Autodesk Fusion 360 part; units mm, degrees
(part 3 of 6)
  spline S86 degree 5 poles (-25.5634, -29.6746) (-25.5637, -29.6656) (-25.5642, -29.6475) (-25.565, -29.6203) (-25.5662, -29.5841) (-25.5679, -29.5389) (-25.5697, -29.4938) (-25.5716, -29.4487) (-25.5738, -29.4036) (-25.576, -29.3586) (-25.5785, -29.3137) (-25.581, -29.2688) (-25.5838, -29.2239) (-25.5867, -29.1791) (-25.5897, -29.1343) (-25.5929, -29.0896) (-25.5963, -29.045) (-25.5998, -29.0004) (-25.6035, -28.9558) (-25.6074, -28.9113) (-25.6114, -28.8669) (-25.6156, -28.8225) (-25.62, -28.7782) (-25.6245, -28.7339) (-25.6292, -28.6897) (-25.6341, -28.6456) (-25.6391, -28.6015) (-25.6443, -28.5575) (-25.6497, -28.5135) (-25.6553, -28.4696) (-25.661, -28.4258) (-25.667, -28.382) (-25.6731, -28.3383) (-25.6794, -28.2947) (-25.6858, -28.2511) (-25.6925, -28.2076) (-25.6993, -28.1642) (-25.7064, -28.1208) (-25.7136, -28.0775) (-25.721, -28.0343) (-25.7287, -27.9912) (-25.7365, -27.9482) (-25.7445, -27.9052) (-25.7527, -27.8623) (-25.7612, -27.8195) (-25.7698, -27.7767) (-25.7773, -27.7409) (-25.7831, -27.7135) (-25.7871, -27.6947) (-25.7894, -27.6845) (-25.7898, -27.6827) knots -1 -1 -1 -1 -1 -1 -0.985714 -0.971429 -0.957143 -0.942857 -0.928571 -0.914286 -0.9 -0.885714 -0.871429 -0.857143 -0.842857 -0.828571 -0.814286 -0.8 -0.785714 -0.771429 -0.757143 -0.742857 -0.728571 -0.714286 -0.7 -0.685714 -0.671429 -0.657143 -0.642857 -0.628571 -0.614286 -0.6 -0.585714 -0.571429 -0.557143 -0.542857 -0.528571 -0.514286 -0.5 -0.485714 -0.471429 -0.457143 -0.442857 -0.428571 -0.414286 -0.4 -0.385714 -0.371429 -0.357143 -0.354152 -0.354152 -0.354152 -0.354152 -0.354152 -0.354152
  spline S87 degree 3 poles (-25.5364, -27.1352) (-25.5938, -27.1658) (-25.6448, -27.2073) (-25.7278, -27.3076) (-25.7591, -27.3654) (-25.7914, -27.4687) (-25.7988, -27.5113) (-25.8026, -27.5975) (-25.7989, -27.6406) (-25.7898, -27.6827) knots 0 0 0 0 0.019532 0.019532 0.039064 0.039064 0.051994 0.051994 0.064924 0.064924 0.064924 0.064924
  arc A44 (-25.5364, -27.1352) -> (-25.4617, -27.0952) centre (-40, 0) ccw
  spline S88 degree 3 poles (-24.8656, -27.1885) (-24.9108, -27.1416) (-24.9648, -27.1041) (-25.084, -27.0518) (-25.1482, -27.0375) (-25.2564, -27.0349) (-25.2994, -27.0394) (-25.3832, -27.0594) (-25.4237, -27.0748) (-25.4617, -27.0952) knots 0 0 0 0 0.019532 0.019532 0.039064 0.039064 0.051994 0.051994 0.064924 0.064924 0.064924 0.064924
  spline S89 degree 5 poles (-24.8656, -27.1885) (-24.8643, -27.1898) (-24.857, -27.1973) (-24.8437, -27.2111) (-24.8242, -27.2311) (-24.7984, -27.2573) (-24.7677, -27.2882) (-24.7368, -27.319) (-24.7057, -27.3496) (-24.6744, -27.3802) (-24.6429, -27.4106) (-24.6113, -27.4409) (-24.5795, -27.471) (-24.5475, -27.5011) (-24.5154, -27.531) (-24.483, -27.5608) (-24.4506, -27.5905) (-24.4179, -27.6201) (-24.3851, -27.6495) (-24.3522, -27.6789) (-24.319, -27.7081) (-24.2858, -27.7372) (-24.2523, -27.7662) (-24.2188, -27.7951) (-24.1851, -27.8239) (-24.1512, -27.8526) (-24.1172, -27.8811) (-24.083, -27.9096) (-24.0487, -27.9379) (-24.0143, -27.9661) (-23.9797, -27.9943) (-23.945, -28.0223) (-23.9101, -28.0502) (-23.8751, -28.078) (-23.84, -28.1057) (-23.8047, -28.1333) (-23.7693, -28.1608) (-23.7338, -28.1882) (-23.6981, -28.2155) (-23.6623, -28.2427) (-23.6264, -28.2697) (-23.5904, -28.2967) (-23.5542, -28.3236) (-23.5179, -28.3504) (-23.4815, -28.377) (-23.4449, -28.4036) (-23.4083, -28.4301) (-23.3788, -28.4512) (-23.3567, -28.4669) (-23.3419, -28.4774) (-23.3345, -28.4827) knots 0.354152 0.354152 0.354152 0.354152 0.354152 0.354152 0.357143 0.371429 0.385714 0.4 0.414286 0.428571 0.442857 0.457143 0.471429 0.485714 0.5 0.514286 0.528571 0.542857 0.557143 0.571429 0.585714 0.6 0.614286 0.628571 0.642857 0.657143 0.671429 0.685714 0.7 0.714286 0.728571 0.742857 0.757143 0.771429 0.785714 0.8 0.814286 0.828571 0.842857 0.857143 0.871429 0.885714 0.9 0.914286 0.928571 0.942857 0.957143 0.971429 0.985714 1 1 1 1 1 1
  arc A45 (-23.3345, -28.4827) -> (-22.7243, -28.1167) centre (-40, 0) ccw
  spline S90 degree 5 poles (-22.7243, -28.1167) (-22.7254, -28.1077) (-22.7277, -28.0897) (-22.7312, -28.0628) (-22.736, -28.0269) (-22.742, -27.9821) (-22.7483, -27.9373) (-22.7546, -27.8927) (-22.7612, -27.848) (-22.7678, -27.8035) (-22.7747, -27.759) (-22.7816, -27.7145) (-22.7887, -27.6701) (-22.796, -27.6258) (-22.8034, -27.5816) (-22.811, -27.5374) (-22.8188, -27.4933) (-22.8266, -27.4493) (-22.8347, -27.4053) (-22.8429, -27.3614) (-22.8513, -27.3176) (-22.8598, -27.2738) (-22.8685, -27.2301) (-22.8773, -27.1865) (-22.8863, -27.143) (-22.8955, -27.0995) (-22.9048, -27.0562) (-22.9143, -27.0129) (-22.924, -26.9696) (-22.9339, -26.9265) (-22.9439, -26.8834) (-22.9541, -26.8405) (-22.9644, -26.7976) (-22.975, -26.7548) (-22.9857, -26.712) (-22.9966, -26.6694) (-23.0076, -26.6268) (-23.0189, -26.5844) (-23.0303, -26.542) (-23.0419, -26.4998) (-23.0538, -26.4576) (-23.0658, -26.4155) (-23.078, -26.3735) (-23.0904, -26.3316) (-23.103, -26.2899) (-23.1158, -26.2482) (-23.1267, -26.2132) (-23.1352, -26.1866) (-23.141, -26.1683) (-23.1443, -26.1583) (-23.1448, -26.1565) knots -1 -1 -1 -1 -1 -1 -0.985714 -0.971429 -0.957143 -0.942857 -0.928571 -0.914286 -0.9 -0.885714 -0.871429 -0.857143 -0.842857 -0.828571 -0.814286 -0.8 -0.785714 -0.771429 -0.757143 -0.742857 -0.728571 -0.714286 -0.7 -0.685714 -0.671429 -0.657143 -0.642857 -0.628571 -0.614286 -0.6 -0.585714 -0.571429 -0.557143 -0.542857 -0.528571 -0.514286 -0.5 -0.485714 -0.471429 -0.457143 -0.442857 -0.428571 -0.414286 -0.4 -0.385714 -0.371429 -0.357143 -0.354152 -0.354152 -0.354152 -0.354152 -0.354152 -0.354152
  spline S91 degree 3 poles (-22.9463, -25.5868) (-23.0005, -25.6229) (-23.0471, -25.6693) (-23.1199, -25.7772) (-23.1454, -25.8378) (-23.1674, -25.9437) (-23.1706, -25.9869) (-23.1659, -26.073) (-23.1581, -26.1155) (-23.1448, -26.1565) knots 0 0 0 0 0.019532 0.019532 0.039064 0.039064 0.051994 0.051994 0.064924 0.064924 0.064924 0.064924
  arc A46 (-22.9463, -25.5868) -> (-22.8759, -25.5397) centre (-40, 0) ccw
  spline S92 degree 3 poles (-22.2735, -25.5741) (-22.3231, -25.5319) (-22.3805, -25.4998) (-22.5043, -25.4595) (-22.5696, -25.4516) (-22.6775, -25.4596) (-22.7199, -25.4683) (-22.8013, -25.4965) (-22.8401, -25.5157) (-22.8759, -25.5397) knots 0 0 0 0 0.019532 0.019532 0.039064 0.039064 0.051994 0.051994 0.064924 0.064924 0.064924 0.064924
  spline S93 degree 5 poles (-22.2735, -25.5741) (-22.2722, -25.5753) (-22.2641, -25.5821) (-22.2495, -25.5945) (-22.2281, -25.6125) (-22.2, -25.636) (-22.1663, -25.6638) (-22.1326, -25.6914) (-22.0986, -25.7188) (-22.0645, -25.7461) (-22.0302, -25.7733) (-21.9957, -25.8004) (-21.9611, -25.8273) (-21.9263, -25.854) (-21.8914, -25.8807) (-21.8563, -25.9072) (-21.8211, -25.9335) (-21.7857, -25.9598) (-21.7502, -25.9859) (-21.7145, -26.0118) (-21.6787, -26.0377) (-21.6427, -26.0634) (-21.6066, -26.089) (-21.5704, -26.1144) (-21.534, -26.1398) (-21.4975, -26.165) (-21.4608, -26.1901) (-21.424, -26.215) (-21.3871, -26.2399) (-21.3501, -26.2646) (-21.3129, -26.2892) (-21.2756, -26.3137) (-21.2382, -26.338) (-21.2006, -26.3623) (-21.163, -26.3864) (-21.1252, -26.4104) (-21.0872, -26.4343) (-21.0492, -26.4581) (-21.011, -26.4817) (-20.9727, -26.5053) (-20.9343, -26.5287) (-20.8958, -26.552) (-20.8572, -26.5752) (-20.8185, -26.5983) (-20.7796, -26.6213) (-20.7406, -26.6441) (-20.7015, -26.6669) (-20.6702, -26.685) (-20.6466, -26.6985) (-20.6309, -26.7075) (-20.623, -26.712) knots 0.354152 0.354152 0.354152 0.354152 0.354152 0.354152 0.357143 0.371429 0.385714 0.4 0.414286 0.428571 0.442857 0.457143 0.471429 0.485714 0.5 0.514286 0.528571 0.542857 0.557143 0.571429 0.585714 0.6 0.614286 0.628571 0.642857 0.657143 0.671429 0.685714 0.7 0.714286 0.728571 0.742857 0.757143 0.771429 0.785714 0.8 0.814286 0.828571 0.842857 0.857143 0.871429 0.885714 0.9 0.914286 0.928571 0.942857 0.957143 0.971429 0.985714 1 1 1 1 1 1
  arc A47 (-20.623, -26.712) -> (-20.0516, -26.288) centre (-40, 0) ccw
  spline S94 degree 5 poles (-20.0516, -26.288) (-20.0536, -26.2792) (-20.0576, -26.2615) (-20.0637, -26.235) (-20.072, -26.1998) (-20.0824, -26.1558) (-20.093, -26.1118) (-20.1037, -26.068) (-20.1146, -26.0242) (-20.1256, -25.9805) (-20.1367, -25.9369) (-20.148, -25.8934) (-20.1595, -25.8499) (-20.1711, -25.8065) (-20.1828, -25.7632) (-20.1947, -25.72) (-20.2067, -25.6769) (-20.2188, -25.6338) (-20.2312, -25.5908) (-20.2436, -25.548) (-20.2562, -25.5052) (-20.269, -25.4625) (-20.2819, -25.4198) (-20.295, -25.3773) (-20.3083, -25.3349) (-20.3216, -25.2925) (-20.3352, -25.2503) (-20.3489, -25.2081) (-20.3628, -25.166) (-20.3768, -25.1241) (-20.391, -25.0822) (-20.4053, -25.0404) (-20.4198, -24.9987) (-20.4345, -24.9572) (-20.4494, -24.9157) (-20.4644, -24.8743) (-20.4796, -24.8331) (-20.4949, -24.7919) (-20.5105, -24.7509) (-20.5262, -24.71) (-20.5421, -24.6692) (-20.5581, -24.6285) (-20.5744, -24.5879) (-20.5908, -24.5474) (-20.6075, -24.5071) (-20.6243, -24.4669) (-20.6386, -24.4331) (-20.6496, -24.4074) (-20.6573, -24.3898) (-20.6615, -24.3802) (-20.6622, -24.3785) knots -1 -1 -1 -1 -1 -1 -0.985714 -0.971429 -0.957143 -0.942857 -0.928571 -0.914286 -0.9 -0.885714 -0.871429 -0.857143 -0.842857 -0.828571 -0.814286 -0.8 -0.785714 -0.771429 -0.757143 -0.742857 -0.728571 -0.714286 -0.7 -0.685714 -0.671429 -0.657143 -0.642857 -0.628571 -0.614286 -0.6 -0.585714 -0.571429 -0.557143 -0.542857 -0.528571 -0.514286 -0.5 -0.485714 -0.471429 -0.457143 -0.442857 -0.428571 -0.414286 -0.4 -0.385714 -0.371429 -0.357143 -0.354152 -0.354152 -0.354152 -0.354152 -0.354152 -0.354152
  spline S95 degree 3 poles (-20.5205, -23.7921) (-20.5709, -23.8333) (-20.6127, -23.884) (-20.6746, -23.9986) (-20.6941, -24.0613) (-20.7055, -24.1689) (-20.7045, -24.2122) (-20.6914, -24.2974) (-20.6794, -24.339) (-20.6622, -24.3785) knots 0 0 0 0 0.019532 0.019532 0.039064 0.039064 0.051994 0.051994 0.064924 0.064924 0.064924 0.064924
  arc A48 (-20.5205, -23.7921) -> (-20.455, -23.7383) centre (-40, 0) ccw
  spline S96 degree 3 poles (-19.8522, -23.7135) (-19.9057, -23.6764) (-19.9659, -23.65) (-20.0931, -23.622) (-20.1588, -23.6205) (-20.2654, -23.6391) (-20.3067, -23.6519) (-20.3851, -23.6879) (-20.4217, -23.7109) (-20.455, -23.7383) knots 0 0 0 0 0.019532 0.019532 0.039064 0.039064 0.051994 0.051994 0.064924 0.064924 0.064924 0.064924
  spline S97 degree 5 poles (-19.8522, -23.7135) (-19.8507, -23.7145) (-19.8421, -23.7205) (-19.8263, -23.7314) (-19.8032, -23.7472) (-19.7729, -23.7678) (-19.7367, -23.7922) (-19.7004, -23.8163) (-19.6639, -23.8403) (-19.6273, -23.8642) (-19.5905, -23.8879) (-19.5535, -23.9114) (-19.5165, -23.9348) (-19.4792, -23.958) (-19.4419, -23.9811) (-19.4043, -24.004) (-19.3667, -24.0268) (-19.3289, -24.0494) (-19.291, -24.0719) (-19.2529, -24.0943) (-19.2148, -24.1165) (-19.1765, -24.1385) (-19.138, -24.1605) (-19.0995, -24.1823) (-19.0608, -24.2039) (-19.022, -24.2254) (-18.983, -24.2468) (-18.944, -24.268) (-18.9048, -24.2891) (-18.8655, -24.3101) (-18.8261, -24.331) (-18.7866, -24.3517) (-18.7469, -24.3722) (-18.7072, -24.3927) (-18.6673, -24.413) (-18.6274, -24.4332) (-18.5873, -24.4533) (-18.5471, -24.4732) (-18.5068, -24.493) (-18.4664, -24.5127) (-18.4259, -24.5322) (-18.3853, -24.5516) (-18.3445, -24.5709) (-18.3037, -24.5901) (-18.2628, -24.6092) (-18.2218, -24.6281) (-18.1807, -24.6469) (-18.1477, -24.6619) (-18.1229, -24.673) (-18.1064, -24.6804) (-18.0981, -24.6841) knots 0.354152 0.354152 0.354152 0.354152 0.354152 0.354152 0.357143 0.371429 0.385714 0.4 0.414286 0.428571 0.442857 0.457143 0.471429 0.485714 0.5 0.514286 0.528571 0.542857 0.557143 0.571429 0.585714 0.6 0.614286 0.628571 0.642857 0.657143 0.671429 0.685714 0.7 0.714286 0.728571 0.742857 0.757143 0.771429 0.785714 0.8 0.814286 0.828571 0.842857 0.857143 0.871429 0.885714 0.9 0.914286 0.928571 0.942857 0.957143 0.971429 0.985714 1 1 1 1 1 1
  arc A49 (-18.0981, -24.6841) -> (-17.5709, -24.2061) centre (-40, 0) ccw
  spline S98 degree 5 poles (-17.5709, -24.2061) (-17.5738, -24.1975) (-17.5796, -24.1804) (-17.5883, -24.1546) (-17.5999, -24.1203) (-17.6146, -24.0776) (-17.6295, -24.0349) (-17.6444, -23.9923) (-17.6595, -23.9498) (-17.6748, -23.9074) (-17.6901, -23.8651) (-17.7056, -23.8229) (-17.7213, -23.7807) (-17.7371, -23.7387) (-17.753, -23.6967) (-17.769, -23.6549) (-17.7852, -23.6131) (-17.8015, -23.5715) (-17.818, -23.5299) (-17.8346, -23.4885) (-17.8514, -23.4471) (-17.8683, -23.4059) (-17.8853, -23.3647) (-17.9025, -23.3237) (-17.9198, -23.2827) (-17.9373, -23.2419) (-17.9549, -23.2012) (-17.9727, -23.1606) (-17.9906, -23.1201) (-18.0087, -23.0797) (-18.0269, -23.0394) (-18.0453, -22.9992) (-18.0638, -22.9592) (-18.0825, -22.9192) (-18.1013, -22.8794) (-18.1203, -22.8397) (-18.1395, -22.8002) (-18.1588, -22.7607) (-18.1783, -22.7214) (-18.1979, -22.6822) (-18.2178, -22.6432) (-18.2377, -22.6042) (-18.2579, -22.5654) (-18.2782, -22.5268) (-18.2987, -22.4883) (-18.3194, -22.4499) (-18.337, -22.4177) (-18.3505, -22.3932) (-18.3598, -22.3764) (-18.3649, -22.3673) (-18.3658, -22.3657) knots -1 -1 -1 -1 -1 -1 -0.985714 -0.971429 -0.957143 -0.942857 -0.928571 -0.914286 -0.9 -0.885714 -0.871429 -0.857143 -0.842857 -0.828571 -0.814286 -0.8 -0.785714 -0.771429 -0.757143 -0.742857 -0.728571 -0.714286 -0.7 -0.685714 -0.671429 -0.657143 -0.642857 -0.628571 -0.614286 -0.6 -0.585714 -0.571429 -0.557143 -0.542857 -0.528571 -0.514286 -0.5 -0.485714 -0.471429 -0.457143 -0.442857 -0.428571 -0.414286 -0.4 -0.385714 -0.371429 -0.357143 -0.354152 -0.354152 -0.354152 -0.354152 -0.354152 -0.354152
  spline S99 degree 3 poles (-18.2823, -21.7682) (-18.3283, -21.8141) (-18.365, -21.8687) (-18.4154, -21.9888) (-18.4286, -22.0532) (-18.4294, -22.1614) (-18.4242, -22.2043) (-18.4028, -22.2878) (-18.3868, -22.328) (-18.3658, -22.3657) knots 0 0 0 0 0.019532 0.019532 0.039064 0.039064 0.051994 0.051994 0.064924 0.064924 0.064924 0.064924
  arc A50 (-18.2823, -21.7682) -> (-18.2224, -21.7082) centre (-40, 0) ccw
  spline S100 degree 3 poles (-17.6249, -21.6244) (-17.6818, -21.5928) (-17.7443, -21.5725) (-17.8736, -21.557) (-17.9391, -21.562) (-18.0434, -21.5909) (-18.0833, -21.6078) (-18.1577, -21.6513) (-18.1919, -21.6777) (-18.2224, -21.7082) knots 0 0 0 0 0.019532 0.019532 0.039064 0.039064 0.051994 0.051994 0.064924 0.064924 0.064924 0.064924
  spline S101 degree 5 poles (-17.6249, -21.6244) (-17.6233, -21.6253) (-17.6141, -21.6305) (-17.5973, -21.6398) (-17.5728, -21.6532) (-17.5407, -21.6708) (-17.5023, -21.6915) (-17.4637, -21.7119) (-17.4251, -21.7322) (-17.3863, -21.7524) (-17.3473, -21.7724) (-17.3083, -21.7922) (-17.2691, -21.8118) (-17.2297, -21.8313) (-17.1903, -21.8506) (-17.1507, -21.8697) (-17.111, -21.8887) (-17.0712, -21.9075) (-17.0313, -21.9262) (-16.9912, -21.9447) (-16.951, -21.963) (-16.9107, -21.9812) (-16.8703, -21.9993) (-16.8298, -22.0172) (-16.7892, -22.035) (-16.7485, -22.0526) (-16.7076, -22.07) (-16.6667, -22.0873) (-16.6256, -22.1045) (-16.5845, -22.1215) (-16.5432, -22.1384) (-16.5018, -22.1551) (-16.4604, -22.1717) (-16.4188, -22.1882) (-16.3772, -22.2045) (-16.3354, -22.2207) (-16.2936, -22.2367) (-16.2516, -22.2526) (-16.2096, -22.2683) (-16.1674, -22.284) (-16.1252, -22.2995) (-16.0829, -22.3148) (-16.0405, -22.33) (-15.9979, -22.3451) (-15.9554, -22.3601) (-15.9127, -22.3749) (-15.8699, -22.3896) (-15.8356, -22.4012) (-15.8099, -22.4099) (-15.7927, -22.4156) (-15.7841, -22.4185) knots 0.354152 0.354152 0.354152 0.354152 0.354152 0.354152 0.357143 0.371429 0.385714 0.4 0.414286 0.428571 0.442857 0.457143 0.471429 0.485714 0.5 0.514286 0.528571 0.542857 0.557143 0.571429 0.585714 0.6 0.614286 0.628571 0.642857 0.657143 0.671429 0.685714 0.7 0.714286 0.728571 0.742857 0.757143 0.771429 0.785714 0.8 0.814286 0.828571 0.842857 0.857143 0.871429 0.885714 0.9 0.914286 0.928571 0.942857 0.957143 0.971429 0.985714 1 1 1 1 1 1
  arc A51 (-15.7841, -22.4185) -> (-15.3063, -21.8912) centre (-40, 0) ccw
  spline S102 degree 5 poles (-15.3063, -21.8912) (-15.31, -21.8829) (-15.3174, -21.8663) (-15.3286, -21.8416) (-15.3436, -21.8086) (-15.3624, -21.7675) (-15.3813, -21.7265) (-15.4004, -21.6855) (-15.4196, -21.6447) (-15.4389, -21.604) (-15.4584, -21.5634) (-15.4779, -21.5229) (-15.4976, -21.4825) (-15.5175, -21.4422) (-15.5374, -21.402) (-15.5575, -21.362) (-15.5777, -21.322) (-15.598, -21.2822) (-15.6185, -21.2424) (-15.6391, -21.2028) (-15.6598, -21.1633) (-15.6807, -21.1239) (-15.7017, -21.0846) (-15.7228, -21.0454) (-15.744, -21.0064) (-15.7654, -20.9675) (-15.787, -20.9287) (-15.8086, -20.89) (-15.8304, -20.8514) (-15.8524, -20.813) (-15.8745, -20.7747) (-15.8967, -20.7365) (-15.919, -20.6985) (-15.9415, -20.6606) (-15.9642, -20.6228) (-15.987, -20.5852) (-16.0099, -20.5477) (-16.033, -20.5103) (-16.0563, -20.4731) (-16.0797, -20.436) (-16.1032, -20.3991) (-16.1269, -20.3623) (-16.1508, -20.3257) (-16.1748, -20.2892) (-16.199, -20.2529) (-16.2233, -20.2167) (-16.244, -20.1864) (-16.2598, -20.1634) (-16.2707, -20.1476) (-16.2767, -20.1389) (-16.2777, -20.1374) knots -1 -1 -1 -1 -1 -1 -0.985714 -0.971429 -0.957143 -0.942857 -0.928571 -0.914286 -0.9 -0.885714 -0.871429 -0.857143 -0.842857 -0.828571 -0.814286 -0.8 -0.785714 -0.771429 -0.757143 -0.742857 -0.728571 -0.714286 -0.7 -0.685714 -0.671429 -0.657143 -0.642857 -0.628571 -0.614286 -0.6 -0.585714 -0.571429 -0.557143 -0.542857 -0.528571 -0.514286 -0.5 -0.485714 -0.471429 -0.457143 -0.442857 -0.428571 -0.414286 -0.4 -0.385714 -0.371429 -0.357143 -0.354152 -0.354152 -0.354152 -0.354152 -0.354152 -0.354152
  spline S103 degree 3 poles (-16.2532, -19.5346) (-16.2945, -19.5849) (-16.3257, -19.6428) (-16.364, -19.7672) (-16.3709, -19.8326) (-16.3611, -19.9404) (-16.3517, -19.9826) (-16.3222, -20.0636) (-16.3023, -20.102) (-16.2777, -20.1374) knots 0 0 0 0 0.019532 0.019532 0.039064 0.039064 0.051994 0.051994 0.064924 0.064924 0.064924 0.064924
  arc A52 (-16.2532, -19.5346) -> (-16.1994, -19.4691) centre (-40, 0) ccw
  spline S104 degree 3 poles (-15.6131, -19.3272) (-15.6728, -19.3012) (-15.737, -19.2872) (-15.8672, -19.2845) (-15.9319, -19.2958) (-16.0328, -19.3348) (-16.0709, -19.3555) (-16.1407, -19.4061) (-16.1722, -19.4358) (-16.1994, -19.4691) knots 0 0 0 0 0.019532 0.019532 0.039064 0.039064 0.051994 0.051994 0.064924 0.064924 0.064924 0.064924
  spline S105 degree 5 poles (-15.6131, -19.3272) (-15.6114, -19.3279) (-15.6018, -19.3321) (-15.5841, -19.3397) (-15.5584, -19.3507) (-15.5247, -19.365) (-15.4845, -19.3818) (-15.4441, -19.3985) (-15.4036, -19.4149) (-15.3631, -19.4311) (-15.3224, -19.4472) (-15.2815, -19.463) (-15.2406, -19.4787) (-15.1996, -19.4943) (-15.1584, -19.5096) (-15.1171, -19.5248) (-15.0758, -19.5398) (-15.0343, -19.5546) (-14.9927, -19.5693) (-14.951, -19.5838) (-14.9093, -19.5981) (-14.8674, -19.6123) (-14.8254, -19.6263) (-14.7833, -19.6401) (-14.7412, -19.6538) (-14.6989, -19.6673) (-14.6565, -19.6807) (-14.6141, -19.6939) (-14.5716, -19.707) (-14.5289, -19.7199) (-14.4862, -19.7326) (-14.4434, -19.7452) (-14.4005, -19.7577) (-14.3576, -19.77) (-14.3145, -19.7821) (-14.2714, -19.7941) (-14.2281, -19.806) (-14.1848, -19.8177) (-14.1414, -19.8292) (-14.098, -19.8407) (-14.0544, -19.8519) (-14.0108, -19.8631) (-13.9671, -19.874) (-13.9233, -19.8849) (-13.8795, -19.8956) (-13.8355, -19.9062) (-13.7915, -19.9166) (-13.7563, -19.9248) (-13.7298, -19.9309) (-13.7121, -19.935) (-13.7033, -19.937) knots 0.354152 0.354152 0.354152 0.354152 0.354152 0.354152 0.357143 0.371429 0.385714 0.4 0.414286 0.428571 0.442857 0.457143 0.471429 0.485714 0.5 0.514286 0.528571 0.542857 0.557143 0.571429 0.585714 0.6 0.614286 0.628571 0.642857 0.657143 0.671429 0.685714 0.7 0.714286 0.728571 0.742857 0.757143 0.771429 0.785714 0.8 0.814286 0.828571 0.842857 0.857143 0.871429 0.885714 0.9 0.914286 0.928571 0.942857 0.957143 0.971429 0.985714 1 1 1 1 1 1
  arc A53 (-13.7033, -19.937) -> (-13.2795, -19.3653) centre (-40, 0) ccw
  spline S106 degree 5 poles (-13.2795, -19.3653) (-13.284, -19.3575) (-13.293, -19.3417) (-13.3066, -19.3182) (-13.3247, -19.2868) (-13.3475, -19.2477) (-13.3703, -19.2088) (-13.3933, -19.1699) (-13.4164, -19.1312) (-13.4396, -19.0926) (-13.463, -19.0541) (-13.4864, -19.0157) (-13.51, -18.9774) (-13.5336, -18.9393) (-13.5574, -18.9012) (-13.5813, -18.8633) (-13.6054, -18.8255) (-13.6295, -18.7879) (-13.6538, -18.7503) (-13.6781, -18.7129) (-13.7026, -18.6756) (-13.7273, -18.6385) (-13.752, -18.6014) (-13.7769, -18.5645) (-13.8018, -18.5277) (-13.827, -18.4911) (-13.8522, -18.4546) (-13.8775, -18.4182) (-13.903, -18.382) (-13.9286, -18.3459) (-13.9543, -18.31) (-13.9802, -18.2741) (-14.0062, -18.2385) (-14.0323, -18.203) (-14.0586, -18.1676) (-14.0849, -18.1324) (-14.1114, -18.0973) (-14.1381, -18.0624) (-14.1649, -18.0276) (-14.1918, -17.993) (-14.2188, -17.9586) (-14.246, -17.9243) (-14.2734, -17.8902) (-14.3008, -17.8562) (-14.3285, -17.8225) (-14.3562, -17.7888) (-14.3797, -17.7607) (-14.3977, -17.7393) (-14.4102, -17.7247) (-14.417, -17.7167) (-14.4182, -17.7153) knots -1 -1 -1 -1 -1 -1 -0.985714 -0.971429 -0.957143 -0.942857 -0.928571 -0.914286 -0.9 -0.885714 -0.871429 -0.857143 -0.842857 -0.828571 -0.814286 -0.8 -0.785714 -0.771429 -0.757143 -0.742857 -0.728571 -0.714286 -0.7 -0.685714 -0.671429 -0.657143 -0.642857 -0.628571 -0.614286 -0.6 -0.585714 -0.571429 -0.557143 -0.542857 -0.528571 -0.514286 -0.5 -0.485714 -0.471429 -0.457143 -0.442857 -0.428571 -0.414286 -0.4 -0.385714 -0.371429 -0.357143 -0.354152 -0.354152 -0.354152 -0.354152 -0.354152 -0.354152
  spline S107 degree 3 poles (-14.4528, -17.113) (-14.489, -17.1671) (-14.5144, -17.2277) (-14.5403, -17.3553) (-14.5407, -17.421) (-14.5204, -17.5273) (-14.5069, -17.5684) (-14.4697, -17.6462) (-14.4461, -17.6825) (-14.4182, -17.7153) knots 0 0 0 0 0.019532 0.019532 0.039064 0.039064 0.051994 0.051994 0.064924 0.064924 0.064924 0.064924
  arc A54 (-14.4528, -17.113) -> (-14.4057, -17.0425) centre (-40, 0) ccw
  spline S108 degree 3 poles (-13.8361, -16.8438) (-13.8981, -16.8238) (-13.9633, -16.8161) (-14.0932, -16.8262) (-14.1565, -16.8438) (-14.2531, -16.8925) (-14.2889, -16.9168) (-14.3534, -16.974) (-14.3819, -17.0066) (-14.4057, -17.0425) knots 0 0 0 0 0.019532 0.019532 0.039064 0.039064 0.051994 0.051994 0.064924 0.064924 0.064924 0.064924
  spline S109 degree 5 poles (-13.8361, -16.8438) (-13.8344, -16.8443) (-13.8244, -16.8476) (-13.8061, -16.8534) (-13.7794, -16.8619) (-13.7444, -16.8728) (-13.7028, -16.8856) (-13.661, -16.8981) (-13.6191, -16.9105) (-13.5771, -16.9227) (-13.535, -16.9347) (-13.4928, -16.9465) (-13.4506, -16.9581) (-13.4082, -16.9695) (-13.3657, -16.9808) (-13.3232, -16.9918) (-13.2806, -17.0027) (-13.2378, -17.0134) (-13.195, -17.0239) (-13.1521, -17.0342) (-13.1091, -17.0444) (-13.0661, -17.0544) (-13.0229, -17.0642) (-12.9797, -17.0739) (-12.9364, -17.0834) (-12.893, -17.0927) (-12.8495, -17.1018) (-12.806, -17.1108) (-12.7624, -17.1196) (-12.7187, -17.1283) (-12.6749, -17.1368) (-12.6311, -17.1452) (-12.5872, -17.1533) (-12.5432, -17.1614) (-12.4992, -17.1692) (-12.4551, -17.177) (-12.4109, -17.1845) (-12.3667, -17.1919) (-12.3223, -17.1992) (-12.278, -17.2063) (-12.2335, -17.2132) (-12.189, -17.22) (-12.1445, -17.2267) (-12.0998, -17.2332) (-12.0551, -17.2395) (-12.0104, -17.2457) (-11.9656, -17.2518) (-11.9297, -17.2565) (-11.9027, -17.26) (-11.8847, -17.2623) (-11.8757, -17.2634) knots 0.354152 0.354152 0.354152 0.354152 0.354152 0.354152 0.357143 0.371429 0.385714 0.4 0.414286 0.428571 0.442857 0.457143 0.471429 0.485714 0.5 0.514286 0.528571 0.542857 0.557143 0.571429 0.585714 0.6 0.614286 0.628571 0.642857 0.657143 0.671429 0.685714 0.7 0.714286 0.728571 0.742857 0.757143 0.771429 0.785714 0.8 0.814286 0.828571 0.842857 0.857143 0.871429 0.885714 0.9 0.914286 0.928571 0.942857 0.957143 0.971429 0.985714 1 1 1 1 1 1
  arc A55 (-11.8757, -17.2634) -> (-11.5101, -16.653) centre (-40, 0) ccw
  spline S110 degree 5 poles (-11.5101, -16.653) (-11.5153, -16.6456) (-11.5258, -16.6309) (-11.5416, -16.6087) (-11.5627, -16.5793) (-11.5892, -16.5427) (-11.6158, -16.5061) (-11.6425, -16.4697) (-11.6692, -16.4334) (-11.6961, -16.3973) (-11.7231, -16.3612) (-11.7502, -16.3253) (-11.7774, -16.2896) (-11.8047, -16.2539) (-11.8321, -16.2184) (-11.8596, -16.183) (-11.8872, -16.1478) (-11.915, -16.1126) (-11.9428, -16.0777) (-11.9707, -16.0428) (-11.9987, -16.0081) (-12.0269, -15.9735) (-12.0551, -15.9391) (-12.0835, -15.9048) (-12.112, -15.8707) (-12.1405, -15.8367) (-12.1692, -15.8028) (-12.198, -15.7691) (-12.2269, -15.7355) (-12.2559, -15.7021) (-12.2851, -15.6689) (-12.3143, -15.6358) (-12.3437, -15.6028) (-12.3731, -15.57) (-12.4027, -15.5374) (-12.4324, -15.5049) (-12.4623, -15.4726) (-12.4922, -15.4405) (-12.5223, -15.4085) (-12.5524, -15.3767) (-12.5827, -15.3451) (-12.6132, -15.3137) (-12.6437, -15.2824) (-12.6744, -15.2513) (-12.7052, -15.2204) (-12.7361, -15.1897) (-12.7623, -15.164) (-12.7823, -15.1445) (-12.7961, -15.1311) (-12.8036, -15.1238) (-12.8049, -15.1225) knots -1 -1 -1 -1 -1 -1 -0.985714 -0.971429 -0.957143 -0.942857 -0.928571 -0.914286 -0.9 -0.885714 -0.871429 -0.857143 -0.842857 -0.828571 -0.814286 -0.8 -0.785714 -0.771429 -0.757143 -0.742857 -0.728571 -0.714286 -0.7 -0.685714 -0.671429 -0.657143 -0.642857 -0.628571 -0.614286 -0.6 -0.585714 -0.571429 -0.557143 -0.542857 -0.528571 -0.514286 -0.5 -0.485714 -0.471429 -0.457143 -0.442857 -0.428571 -0.414286 -0.4 -0.385714 -0.371429 -0.357143 -0.354152 -0.354152 -0.354152 -0.354152 -0.354152 -0.354152
  spline S111 degree 3 poles (-12.8985, -14.5265) (-12.9292, -14.5839) (-12.9485, -14.6467) (-12.9618, -14.7763) (-12.9558, -14.8417) (-12.9251, -14.9455) (-12.9077, -14.9851) (-12.863, -15.0588) (-12.836, -15.0926) (-12.8049, -15.1225) knots 0 0 0 0 0.019532 0.019532 0.039064 0.039064 0.051994 0.051994 0.064924 0.064924 0.064924 0.064924
  arc A56 (-12.8985, -14.5265) -> (-12.8585, -14.4518) centre (-40, 0) ccw
  spline S112 degree 3 poles (-12.3111, -14.1982) (-12.3747, -14.1843) (-12.4405, -14.1831) (-12.5687, -14.2058) (-12.6299, -14.2296) (-12.7213, -14.2876) (-12.7546, -14.3153) (-12.8132, -14.3785) (-12.8383, -14.4137) (-12.8585, -14.4518) knots 0 0 0 0 0.019532 0.019532 0.039064 0.039064 0.051994 0.051994 0.064924 0.064924 0.064924 0.064924
  spline S113 degree 5 poles (-12.3111, -14.1982) (-12.3093, -14.1985) (-12.2991, -14.2008) (-12.2803, -14.2048) (-12.2529, -14.2106) (-12.217, -14.2181) (-12.1743, -14.2267) (-12.1315, -14.2351) (-12.0886, -14.2433) (-12.0456, -14.2513) (-12.0026, -14.2591) (-11.9594, -14.2667) (-11.9162, -14.2741) (-11.8729, -14.2814) (-11.8296, -14.2884) (-11.7862, -14.2952) (-11.7427, -14.3018) (-11.6991, -14.3083) (-11.6554, -14.3146) (-11.6117, -14.3207) (-11.568, -14.3266) (-11.5241, -14.3323) (-11.4802, -14.3378) (-11.4363, -14.3432) (-11.3922, -14.3484) (-11.3481, -14.3534) (-11.304, -14.3583) (-11.2598, -14.3629) (-11.2155, -14.3675) (-11.1712, -14.3718) (-11.1268, -14.376) (-11.0824, -14.38) (-11.0379, -14.3838) (-10.9933, -14.3875) (-10.9487, -14.391) (-10.9041, -14.3944) (-10.8594, -14.3976) (-10.8146, -14.4006) (-10.7698, -14.4035) (-10.725, -14.4062) (-10.68, -14.4088) (-10.6351, -14.4112) (-10.5901, -14.4134) (-10.545, -14.4155) (-10.4999, -14.4174) (-10.4548, -14.4192) (-10.4096, -14.4209) (-10.3734, -14.4221) (-10.3462, -14.4229) (-10.3281, -14.4234) (-10.3191, -14.4236) knots 0.354152 0.354152 0.354152 0.354152 0.354152 0.354152 0.357143 0.371429 0.385714 0.4 0.414286 0.428571 0.442857 0.457143 0.471429 0.485714 0.5 0.514286 0.528571 0.542857 0.557143 0.571429 0.585714 0.6 0.614286 0.628571 0.642857 0.657143 0.671429 0.685714 0.7 0.714286 0.728571 0.742857 0.757143 0.771429 0.785714 0.8 0.814286 0.828571 0.842857 0.857143 0.871429 0.885714 0.9 0.914286 0.928571 0.942857 0.957143 0.971429 0.985714 1 1 1 1 1 1
  arc A57 (-10.3191, -14.4236) -> (-10.015, -13.7803) centre (-40, 0) ccw
  spline S114 degree 5 poles (-10.015, -13.7803) (-10.0209, -13.7735) (-10.0328, -13.7598) (-10.0507, -13.7393) (-10.0746, -13.7121) (-10.1045, -13.6783) (-10.1346, -13.6445) (-10.1647, -13.6109) (-10.1949, -13.5774) (-10.2252, -13.5441) (-10.2556, -13.5108) (-10.2861, -13.4778) (-10.3167, -13.4448) (-10.3473, -13.412) (-10.3781, -13.3794) (-10.4089, -13.3468) (-10.4399, -13.3145) (-10.4709, -13.2822) (-10.502, -13.2501) (-10.5332, -13.2182) (-10.5645, -13.1864) (-10.5959, -13.1548) (-10.6274, -13.1233) (-10.659, -13.0919) (-10.6907, -13.0607) (-10.7224, -13.0297) (-10.7543, -12.9988) (-10.7862, -12.9681) (-10.8183, -12.9375) (-10.8505, -12.9071) (-10.8827, -12.8769) (-10.9151, -12.8468) (-10.9475, -12.8169) (-10.98, -12.7872) (-11.0127, -12.7576) (-11.0454, -12.7282) (-11.0783, -12.699) (-11.1112, -12.6699) (-11.1443, -12.641) (-11.1774, -12.6124) (-11.2107, -12.5839) (-11.244, -12.5555) (-11.2775, -12.5274) (-11.3111, -12.4995) (-11.3448, -12.4717) (-11.3785, -12.4442) (-11.4071, -12.4212) (-11.4289, -12.4037) (-11.444, -12.3918) (-11.4522, -12.3853) (-11.4536, -12.3841) knots -1 -1 -1 -1 -1 -1 -0.985714 -0.971429 -0.957143 -0.942857 -0.928571 -0.914286 -0.9 -0.885714 -0.871429 -0.857143 -0.842857 -0.828571 -0.814286 -0.8 -0.785714 -0.771429 -0.757143 -0.742857 -0.728571 -0.714286 -0.7 -0.685714 -0.671429 -0.657143 -0.642857 -0.628571 -0.614286 -0.6 -0.585714 -0.571429 -0.557143 -0.542857 -0.528571 -0.514286 -0.5 -0.485714 -0.471429 -0.457143 -0.442857 -0.428571 -0.414286 -0.4 -0.385714 -0.371429 -0.357143 -0.354152 -0.354152 -0.354152 -0.354152 -0.354152 -0.354152
  spline S115 degree 3 poles (-11.6051, -11.8001) (-11.6301, -11.8603) (-11.6431, -11.9247) (-11.6437, -12.0549) (-11.6312, -12.1194) (-11.5906, -12.2197) (-11.5693, -12.2574) (-11.5176, -12.3264) (-11.4874, -12.3574) (-11.4536, -12.3841) knots 0 0 0 0 0.019532 0.019532 0.039064 0.039064 0.051994 0.051994 0.064924 0.064924 0.064924 0.064924
  arc A58 (-11.6051, -11.8001) -> (-11.5727, -11.7219) centre (-40, 0) ccw
  spline S116 degree 3 poles (-11.0528, -11.4158) (-11.1175, -11.4083) (-11.183, -11.4135) (-11.3083, -11.4487) (-11.367, -11.4784) (-11.4522, -11.545) (-11.4826, -11.5758) (-11.5348, -11.6445) (-11.5563, -11.682) (-11.5727, -11.7219) knots 0 0 0 0 0.019532 0.019532 0.039064 0.039064 0.051994 0.051994 0.064924 0.064924 0.064924 0.064924
  spline S117 degree 5 poles (-11.0528, -11.4158) (-11.051, -11.416) (-11.0405, -11.4172) (-11.0214, -11.4194) (-10.9937, -11.4225) (-10.9572, -11.4264) (-10.9138, -11.4308) (-10.8704, -11.435) (-10.8269, -11.4389) (-10.7834, -11.4427) (-10.7397, -11.4462) (-10.6961, -11.4496) (-10.6524, -11.4527) (-10.6086, -11.4557) (-10.5647, -11.4584) (-10.5208, -11.4609) (-10.4769, -11.4633) (-10.4329, -11.4654) (-10.3889, -11.4674) (-10.3448, -11.4692) (-10.3006, -11.4707) (-10.2564, -11.4721) (-10.2122, -11.4734) (-10.1679, -11.4744) (-10.1236, -11.4753) (-10.0792, -11.4759) (-10.0348, -11.4764) (-9.9904, -11.4768) (-9.9459, -11.4769) (-9.9013, -11.4769) (-9.8568, -11.4767) (-9.8121, -11.4763) (-9.7675, -11.4758) (-9.7228, -11.4751) (-9.6781, -11.4742) (-9.6333, -11.4732) (-9.5885, -11.472) (-9.5436, -11.4706) (-9.4988, -11.4691) (-9.4539, -11.4674) (-9.4089, -11.4655) (-9.3639, -11.4635) (-9.3189, -11.4613) (-9.2739, -11.459) (-9.2288, -11.4565) (-9.1837, -11.4539) (-9.1386, -11.4511) (-9.1025, -11.4487) (-9.0753, -11.4469) (-9.0573, -11.4456) (-9.0482, -11.445) knots 0.354152 0.354152 0.354152 0.354152 0.354152 0.354152 0.357143 0.371429 0.385714 0.4 0.414286 0.428571 0.442857 0.457143 0.471429 0.485714 0.5 0.514286 0.528571 0.542857 0.557143 0.571429 0.585714 0.6 0.614286 0.628571 0.642857 0.657143 0.671429 0.685714 0.7 0.714286 0.728571 0.742857 0.757143 0.771429 0.785714 0.8 0.814286 0.828571 0.842857 0.857143 0.871429 0.885714 0.9 0.914286 0.928571 0.942857 0.957143 0.971429 0.985714 1 1 1 1 1 1
  arc A59 (-9.0482, -11.445) -> (-8.8086, -10.7749) centre (-40, 0) ccw
  spline S118 degree 5 poles (-8.8086, -10.7749) (-8.8152, -10.7687) (-8.8284, -10.7563) (-8.8482, -10.7376) (-8.8746, -10.7129) (-8.9078, -10.6821) (-8.941, -10.6515) (-8.9743, -10.621) (-9.0076, -10.5906) (-9.041, -10.5604) (-9.0745, -10.5303) (-9.1081, -10.5004) (-9.1418, -10.4706) (-9.1755, -10.441) (-9.2093, -10.4115) (-9.2432, -10.3821) (-9.2771, -10.353) (-9.3112, -10.3239) (-9.3453, -10.295) (-9.3795, -10.2663) (-9.4138, -10.2377) (-9.4481, -10.2093) (-9.4825, -10.1811) (-9.517, -10.153) (-9.5516, -10.125) (-9.5863, -10.0972) (-9.621, -10.0696) (-9.6558, -10.0422) (-9.6907, -10.0149) (-9.7257, -9.9878) (-9.7608, -9.9609) (-9.7959, -9.9341) (-9.8311, -9.9075) (-9.8664, -9.8811) (-9.9018, -9.8549) (-9.9373, -9.8288) (-9.9728, -9.803) (-10.0085, -9.7773) (-10.0442, -9.7518) (-10.08, -9.7265) (-10.1159, -9.7014) (-10.1518, -9.6765) (-10.1879, -9.6518) (-10.2241, -9.6273) (-10.2603, -9.603) (-10.2966, -9.5789) (-10.3273, -9.5588) (-10.3507, -9.5436) (-10.3669, -9.5331) (-10.3757, -9.5274) (-10.3772, -9.5265) knots -1 -1 -1 -1 -1 -1 -0.985714 -0.971429 -0.957143 -0.942857 -0.928571 -0.914286 -0.9 -0.885714 -0.871429 -0.857143 -0.842857 -0.828571 -0.814286 -0.8 -0.785714 -0.771429 -0.757143 -0.742857 -0.728571 -0.714286 -0.7 -0.685714 -0.671429 -0.657143 -0.642857 -0.628571 -0.614286 -0.6 -0.585714 -0.571429 -0.557143 -0.542857 -0.528571 -0.514286 -0.5 -0.485714 -0.471429 -0.457143 -0.442857 -0.428571 -0.414286 -0.4 -0.385714 -0.371429 -0.357143 -0.354152 -0.354152 -0.354152 -0.354152 -0.354152 -0.354152
  spline S119 degree 3 poles (-10.5852, -8.9601) (-10.6042, -9.0224) (-10.6108, -9.0878) (-10.5986, -9.2174) (-10.5799, -9.2805) (-10.5297, -9.3763) (-10.5048, -9.4117) (-10.4466, -9.4753) (-10.4135, -9.5032) (-10.3772, -9.5265) knots 0 0 0 0 0.019532 0.019532 0.039064 0.039064 0.051994 0.051994 0.064924 0.064924 0.064924 0.064924
  arc A60 (-10.5852, -8.9601) -> (-10.5606, -8.8791) centre (-40, 0) ccw
  spline S120 degree 3 poles (-10.0732, -8.5235) (-10.1383, -8.5224) (-10.203, -8.534) (-10.3243, -8.5813) (-10.3798, -8.6166) (-10.4581, -8.6912) (-10.4853, -8.7249) (-10.5305, -8.7983) (-10.5482, -8.8378) (-10.5606, -8.8791) knots 0 0 0 0 0.019532 0.019532 0.039064 0.039064 0.051994 0.051994 0.064924 0.064924 0.064924 0.064924
  spline S121 degree 5 poles (-10.0732, -8.5235) (-10.0714, -8.5235) (-10.0609, -8.5237) (-10.0417, -8.524) (-10.0137, -8.5244) (-9.9771, -8.5247) (-9.9335, -8.5248) (-9.8899, -8.5247) (-9.8462, -8.5244) (-9.8025, -8.5239) (-9.7587, -8.5231) (-9.7149, -8.5222) (-9.6711, -8.521) (-9.6272, -8.5196) (-9.5834, -8.5181) (-9.5394, -8.5163) (-9.4955, -8.5143) (-9.4515, -8.5121) (-9.4074, -8.5098) (-9.3634, -8.5072) (-9.3193, -8.5045) (-9.2752, -8.5015) (-9.2311, -8.4984) (-9.1869, -8.4951) (-9.1427, -8.4916) (-9.0985, -8.4879) (-9.0542, -8.4841) (-9.01, -8.48) (-8.9657, -8.4758) (-8.9213, -8.4714) (-8.877, -8.4669) (-8.8326, -8.4621) (-8.7882, -8.4572) (-8.7438, -8.4521) (-8.6994, -8.4469) (-8.6549, -8.4415) (-8.6105, -8.4359) (-8.566, -8.4301) (-8.5215, -8.4242) (-8.477, -8.4181) (-8.4324, -8.4119) (-8.3878, -8.4054) (-8.3433, -8.3989) (-8.2987, -8.3921) (-8.2541, -8.3852) (-8.2094, -8.3782) (-8.1648, -8.371) (-8.1291, -8.3651) (-8.1023, -8.3606) (-8.0844, -8.3576) (-8.0755, -8.356) knots 0.354152 0.354152 0.354152 0.354152 0.354152 0.354152 0.357143 0.371429 0.385714 0.4 0.414286 0.428571 0.442857 0.457143 0.471429 0.485714 0.5 0.514286 0.528571 0.542857 0.557143 0.571429 0.585714 0.6 0.614286 0.628571 0.642857 0.657143 0.671429 0.685714 0.7 0.714286 0.728571 0.742857 0.757143 0.771429 0.785714 0.8 0.814286 0.828571 0.842857 0.857143 0.871429 0.885714 0.9 0.914286 0.928571 0.942857 0.957143 0.971429 0.985714 1 1 1 1 1 1
  arc A61 (-8.0755, -8.356) -> (-7.9027, -7.6658) centre (-40, 0) ccw
  spline S122 degree 5 poles (-7.9027, -7.6658) (-7.9099, -7.6602) (-7.9242, -7.6491) (-7.9457, -7.6325) (-7.9745, -7.6105) (-8.0105, -7.5831) (-8.0465, -7.5559) (-8.0826, -7.5288) (-8.1188, -7.5018) (-8.155, -7.475) (-8.1913, -7.4484) (-8.2276, -7.4219) (-8.2641, -7.3956) (-8.3005, -7.3694) (-8.3371, -7.3433) (-8.3737, -7.3175) (-8.4103, -7.2917) (-8.447, -7.2662) (-8.4838, -7.2408) (-8.5207, -7.2155) (-8.5576, -7.1905) (-8.5945, -7.1655) (-8.6316, -7.1408) (-8.6686, -7.1162) (-8.7058, -7.0918) (-8.743, -7.0676) (-8.7803, -7.0435) (-8.8176, -7.0196) (-8.855, -6.9959) (-8.8925, -6.9723) (-8.93, -6.949) (-8.9676, -6.9258) (-9.0053, -6.9028) (-9.043, -6.8799) (-9.0808, -6.8573) (-9.1186, -6.8349) (-9.1566, -6.8126) (-9.1945, -6.7905) (-9.2326, -6.7687) (-9.2707, -6.747) (-9.3089, -6.7255) (-9.3471, -6.7043) (-9.3854, -6.6832) (-9.4238, -6.6624) (-9.4622, -6.6417) (-9.5008, -6.6213) (-9.5332, -6.6043) (-9.558, -6.5915) (-9.5751, -6.5827) (-9.5845, -6.5779) (-9.5861, -6.5771) knots -1 -1 -1 -1 -1 -1 -0.985714 -0.971429 -0.957143 -0.942857 -0.928571 -0.914286 -0.9 -0.885714 -0.871429 -0.857143 -0.842857 -0.828571 -0.814286 -0.8 -0.785714 -0.771429 -0.757143 -0.742857 -0.728571 -0.714286 -0.7 -0.685714 -0.671429 -0.657143 -0.642857 -0.628571 -0.614286 -0.6 -0.585714 -0.571429 -0.557143 -0.542857 -0.528571 -0.514286 -0.5 -0.485714 -0.471429 -0.457143 -0.442857 -0.428571 -0.414286 -0.4 -0.385714 -0.371429 -0.357143 -0.354152 -0.354152 -0.354152 -0.354152 -0.354152 -0.354152
  spline S123 degree 3 poles (-9.8486, -6.0338) (-9.8614, -6.0977) (-9.8616, -6.1634) (-9.8367, -6.2912) (-9.812, -6.3521) (-9.7525, -6.4425) (-9.7243, -6.4753) (-9.6601, -6.5329) (-9.6245, -6.5574) (-9.5861, -6.5771) knots 0 0 0 0 0.019532 0.019532 0.039064 0.039064 0.051994 0.051994 0.064924 0.064924 0.064924 0.064924
  arc A62 (-9.8486, -6.0338) -> (-9.8321, -5.9507) centre (-40, 0) ccw
  spline S124 degree 3 poles (-9.3819, -5.5491) (-9.4468, -5.5544) (-9.51, -5.5723) (-9.6261, -5.6312) (-9.6778, -5.6718) (-9.7485, -5.7538) (-9.7723, -5.7899) (-9.81, -5.8674) (-9.8238, -5.9085) (-9.8321, -5.9507) knots 0 0 0 0 0.019532 0.019532 0.039064 0.039064 0.051994 0.051994 0.064924 0.064924 0.064924 0.064924
  spline S125 degree 5 poles (-9.3819, -5.5491) (-9.3801, -5.549) (-9.3696, -5.5481) (-9.3504, -5.5465) (-9.3226, -5.5442) (-9.2861, -5.5409) (-9.2427, -5.5367) (-9.1993, -5.5323) (-9.1558, -5.5277) (-9.1124, -5.5229) (-9.0689, -5.5179) (-9.0254, -5.5127) (-8.9819, -5.5072) (-8.9384, -5.5015) (-8.8949, -5.4957) (-8.8514, -5.4896) (-8.8078, -5.4833) (-8.7642, -5.4769) (-8.7207, -5.4702) (-8.6771, -5.4633) (-8.6335, -5.4563) (-8.5898, -5.449) (-8.5462, -5.4416) (-8.5026, -5.434) (-8.459, -5.4262) (-8.4153, -5.4182) (-8.3717, -5.41) (-8.328, -5.4016) (-8.2843, -5.3931) (-8.2406, -5.3844) (-8.197, -5.3755) (-8.1533, -5.3664) (-8.1096, -5.3572) (-8.0659, -5.3478) (-8.0222, -5.3382) (-7.9785, -5.3285) (-7.9348, -5.3185) (-7.8911, -5.3084) (-7.8473, -5.2982) (-7.8036, -5.2878) (-7.7599, -5.2772) (-7.7162, -5.2664) (-7.6725, -5.2555) (-7.6287, -5.2444) (-7.585, -5.2332) (-7.5413, -5.2218) (-7.4976, -5.2103) (-7.4626, -5.2009) (-7.4364, -5.1938) (-7.4189, -5.189) (-7.4101, -5.1866) knots 0.354152 0.354152 0.354152 0.354152 0.354152 0.354152 0.357143 0.371429 0.385714 0.4 0.414286 0.428571 0.442857 0.457143 0.471429 0.485714 0.5 0.514286 0.528571 0.542857 0.557143 0.571429 0.585714 0.6 0.614286 0.628571 0.642857 0.657143 0.671429 0.685714 0.7 0.714286 0.728571 0.742857 0.757143 0.771429 0.785714 0.8 0.814286 0.828571 0.842857 0.857143 0.871429 0.885714 0.9 0.914286 0.928571 0.942857 0.957143 0.971429 0.985714 1 1 1 1 1 1
  arc A63 (-7.4101, -5.1866) -> (-7.3059, -4.4828) centre (-40, 0) ccw
  spline S126 degree 5 poles (-7.3059, -4.4828) (-7.3136, -4.4779) (-7.3289, -4.4683) (-7.352, -4.4539) (-7.3827, -4.4348) (-7.4212, -4.4111) (-7.4598, -4.3875) (-7.4984, -4.3641) (-7.537, -4.3408) (-7.5757, -4.3177) (-7.6144, -4.2947) (-7.6532, -4.2719) (-7.692, -4.2493) (-7.7308, -4.2268) (-7.7698, -4.2045) (-7.8087, -4.1823) (-7.8477, -4.1603) (-7.8868, -4.1385) (-7.9259, -4.1168) (-7.965, -4.0953) (-8.0042, -4.0739) (-8.0434, -4.0528) (-8.0827, -4.0318) (-8.122, -4.0109) (-8.1614, -3.9903) (-8.2008, -3.9698) (-8.2402, -3.9495) (-8.2797, -3.9294) (-8.3193, -3.9094) (-8.3589, -3.8897) (-8.3985, -3.8701) (-8.4382, -3.8507) (-8.4779, -3.8315) (-8.5177, -3.8125) (-8.5575, -3.7937) (-8.5974, -3.775) (-8.6373, -3.7566) (-8.6773, -3.7384) (-8.7173, -3.7203) (-8.7573, -3.7025) (-8.7974, -3.6849) (-8.8376, -3.6675) (-8.8778, -3.6503) (-8.918, -3.6333) (-8.9583, -3.6165) (-8.9986, -3.6) (-9.0326, -3.5862) (-9.0586, -3.5759) (-9.0764, -3.5688) (-9.0862, -3.565) (-9.0879, -3.5643) knots -1 -1 -1 -1 -1 -1 -0.985714 -0.971429 -0.957143 -0.942857 -0.928571 -0.914286 -0.9 -0.885714 -0.871429 -0.857143 -0.842857 -0.828571 -0.814286 -0.8 -0.785714 -0.771429 -0.757143 -0.742857 -0.728571 -0.714286 -0.7 -0.685714 -0.671429 -0.657143 -0.642857 -0.628571 -0.614286 -0.6 -0.585714 -0.571429 -0.557143 -0.542857 -0.528571 -0.514286 -0.5 -0.485714 -0.471429 -0.457143 -0.442857 -0.428571 -0.414286 -0.4 -0.385714 -0.371429 -0.357143 -0.354152 -0.354152 -0.354152 -0.354152 -0.354152 -0.354152
  spline S127 degree 3 poles (-9.4024, -3.0494) (-9.4088, -3.1142) (-9.4026, -3.1796) (-9.3653, -3.3044) (-9.3347, -3.3626) (-9.2667, -3.4467) (-9.2354, -3.4766) (-9.1659, -3.5276) (-9.128, -3.5485) (-9.0879, -3.5643) knots 0 0 0 0 0.019532 0.019532 0.039064 0.039064 0.051994 0.051994 0.064924 0.064924 0.064924 0.064924
  arc A64 (-9.4024, -3.0494) -> (-9.3941, -2.9651) centre (-40, 0) ccw
  spline S128 degree 3 poles (-8.9854, -2.5213) (-9.0495, -2.5329) (-9.1107, -2.5569) (-9.2204, -2.627) (-9.2679, -2.6724) (-9.3302, -2.7609) (-9.3503, -2.7992) (-9.3803, -2.88) (-9.3899, -2.9222) (-9.3941, -2.9651) knots 0 0 0 0 0.019532 0.019532 0.039064 0.039064 0.051994 0.051994 0.064924 0.064924 0.064924 0.064924
  spline S129 degree 5 poles (-8.9854, -2.5213) (-8.9836, -2.521) (-8.9733, -2.5191) (-8.9544, -2.5157) (-8.9269, -2.5105) (-8.8909, -2.5037) (-8.8481, -2.4953) (-8.8053, -2.4867) (-8.7626, -2.4779) (-8.7198, -2.4688) (-8.677, -2.4596) (-8.6343, -2.4501) (-8.5915, -2.4404) (-8.5488, -2.4305) (-8.506, -2.4204) (-8.4633, -2.4101) (-8.4205, -2.3996) (-8.3778, -2.3889) (-8.3351, -2.3779) (-8.2924, -2.3668) (-8.2497, -2.3555) (-8.207, -2.3441) (-8.1643, -2.3324) (-8.1216, -2.3205) (-8.079, -2.3085) (-8.0363, -2.2962) (-7.9937, -2.2838) (-7.951, -2.2712) (-7.9084, -2.2585) (-7.8658, -2.2455) (-7.8232, -2.2324) (-7.7806, -2.2191) (-7.738, -2.2056) (-7.6955, -2.192) (-7.6529, -2.1781) (-7.6104, -2.1641) (-7.5679, -2.15) (-7.5254, -2.1357) (-7.4829, -2.1212) (-7.4404, -2.1065) (-7.3979, -2.0917) (-7.3554, -2.0767) (-7.313, -2.0616) (-7.2706, -2.0463) (-7.2282, -2.0308) (-7.1858, -2.0152) (-7.1434, -1.9994) (-7.1095, -1.9866) (-7.0841, -1.977) (-7.0672, -1.9705) (-7.0587, -1.9673) knots 0.354152 0.354152 0.354152 0.354152 0.354152 0.354152 0.357143 0.371429 0.385714 0.4 0.414286 0.428571 0.442857 0.457143 0.471429 0.485714 0.5 0.514286 0.528571 0.542857 0.557143 0.571429 0.585714 0.6 0.614286 0.628571 0.642857 0.657143 0.671429 0.685714 0.7 0.714286 0.728571 0.742857 0.757143 0.771429 0.785714 0.8 0.814286 0.828571 0.842857 0.857143 0.871429 0.885714 0.9 0.914286 0.928571 0.942857 0.957143 0.971429 0.985714 1 1 1 1 1 1
  arc A65 (-7.0587, -1.9673) -> (-7.0239, -1.2566) centre (-40, 0) ccw
  spline S130 degree 5 poles (-7.0239, -1.2566) (-7.032, -1.2525) (-7.0483, -1.2445) (-7.0726, -1.2324) (-7.1051, -1.2164) (-7.1457, -1.1966) (-7.1864, -1.1769) (-7.2271, -1.1573) (-7.2678, -1.138) (-7.3086, -1.1188) (-7.3494, -1.0997) (-7.3902, -1.0808) (-7.4311, -1.0621) (-7.4719, -1.0435) (-7.5128, -1.0251) (-7.5538, -1.0069) (-7.5948, -0.9888) (-7.6358, -0.9709) (-7.6768, -0.9531) (-7.7178, -0.9356) (-7.7589, -0.9182) (-7.8, -0.901) (-7.8412, -0.8839) (-7.8824, -0.867) (-7.9236, -0.8503) (-7.9648, -0.8338) (-8.0061, -0.8175) (-8.0473, -0.8013) (-8.0887, -0.7854) (-8.13, -0.7696) (-8.1714, -0.754) (-8.2128, -0.7386) (-8.2542, -0.7234) (-8.2956, -0.7083) (-8.3371, -0.6935) (-8.3786, -0.6789) (-8.4201, -0.6644) (-8.4617, -0.6502) (-8.5033, -0.6362) (-8.5449, -0.6224) (-8.5865, -0.6088) (-8.6282, -0.5954) (-8.6698, -0.5822) (-8.7115, -0.5692) (-8.7533, -0.5565) (-8.795, -0.544) (-8.8302, -0.5336) (-8.857, -0.5259) (-8.8755, -0.5206) (-8.8856, -0.5177) (-8.8874, -0.5172) knots -1 -1 -1 -1 -1 -1 -0.985714 -0.971429 -0.957143 -0.942857 -0.928571 -0.914286 -0.9 -0.885714 -0.871429 -0.857143 -0.842857 -0.828571 -0.814286 -0.8 -0.785714 -0.771429 -0.757143 -0.742857 -0.728571 -0.714286 -0.7 -0.685714 -0.671429 -0.657143 -0.642857 -0.628571 -0.614286 -0.6 -0.585714 -0.571429 -0.557143 -0.542857 -0.528571 -0.514286 -0.5 -0.485714 -0.471429 -0.457143 -0.442857 -0.428571 -0.414286 -0.4 -0.385714 -0.371429 -0.357143 -0.354152 -0.354152 -0.354152 -0.354152 -0.354152 -0.354152
  spline S131 degree 3 poles (-9.2508, -0.0357) (-9.2509, -0.1008) (-9.2383, -0.1653) (-9.189, -0.2858) (-9.1528, -0.3407) (-9.0769, -0.4178) (-9.0428, -0.4444) (-8.9686, -0.4884) (-8.9288, -0.5054) (-8.8874, -0.5172) knots 0 0 0 0 0.019532 0.019532 0.039064 0.039064 0.051994 0.051994 0.064924 0.064924 0.064924 0.064924
  arc A66 (-9.2508, -0.0357) -> (-9.2508, 0.0491) centre (-40, 0) ccw
  spline S132 degree 3 poles (-8.8876, 0.5308) (-8.9502, 0.513) (-9.0088, 0.4831) (-9.1111, 0.4026) (-9.154, 0.3527) (-9.2072, 0.2586) (-9.2235, 0.2185) (-9.2454, 0.1351) (-9.2509, 0.0922) (-9.2508, 0.0491) knots 0 0 0 0 0.019532 0.019532 0.039064 0.039064 0.051994 0.051994 0.064924 0.064924 0.064924 0.064924
  spline S133 degree 5 poles (-8.8876, 0.5308) (-8.8859, 0.5313) (-8.8758, 0.5342) (-8.8573, 0.5395) (-8.8304, 0.5472) (-8.7953, 0.5576) (-8.7535, 0.5701) (-8.7118, 0.5829) (-8.6701, 0.5959) (-8.6284, 0.6091) (-8.5868, 0.6225) (-8.5451, 0.6361) (-8.5035, 0.6499) (-8.462, 0.664) (-8.4204, 0.6782) (-8.3789, 0.6927) (-8.3374, 0.7073) (-8.2959, 0.7222) (-8.2545, 0.7372) (-8.2131, 0.7524) (-8.1717, 0.7679) (-8.1303, 0.7835) (-8.089, 0.7993) (-8.0477, 0.8153) (-8.0064, 0.8314) (-7.9652, 0.8478) (-7.9239, 0.8643) (-7.8827, 0.8811) (-7.8416, 0.8979) (-7.8004, 0.915) (-7.7593, 0.9322) (-7.7183, 0.9497) (-7.6772, 0.9672) (-7.6362, 0.985) (-7.5952, 1.0029) (-7.5542, 1.021) (-7.5133, 1.0393) (-7.4724, 1.0577) (-7.4315, 1.0763) (-7.3907, 1.095) (-7.3499, 1.1139) (-7.3091, 1.133) (-7.2683, 1.1522) (-7.2276, 1.1716) (-7.1869, 1.1912) (-7.1463, 1.2109) (-7.1056, 1.2308) (-7.0732, 1.2468) (-7.0488, 1.2588) (-7.0326, 1.2669) (-7.0245, 1.271) knots 0.354152 0.354152 0.354152 0.354152 0.354152 0.354152 0.357143 0.371429 0.385714 0.4 0.414286 0.428571 0.442857 0.457143 0.471429 0.485714 0.5 0.514286 0.528571 0.542857 0.557143 0.571429 0.585714 0.6 0.614286 0.628571 0.642857 0.657143 0.671429 0.685714 0.7 0.714286 0.728571 0.742857 0.757143 0.771429 0.785714 0.8 0.814286 0.828571 0.842857 0.857143 0.871429 0.885714 0.9 0.914286 0.928571 0.942857 0.957143 0.971429 0.985714 1 1 1 1 1 1
  arc A67 (-7.0245, 1.271) -> (-7.0596, 1.9817) centre (-40, 0) ccw
  spline S134 degree 5 poles (-7.0596, 1.9817) (-7.068, 1.9849) (-7.085, 1.9914) (-7.1104, 2.001) (-7.1443, 2.0137) (-7.1867, 2.0295) (-7.2291, 2.0451) (-7.2715, 2.0605) (-7.3139, 2.0758) (-7.3564, 2.091) (-7.3988, 2.1059) (-7.4413, 2.1207) (-7.4838, 2.1354) (-7.5263, 2.1498) (-7.5688, 2.1641) (-7.6113, 2.1783) (-7.6539, 2.1922) (-7.6964, 2.206) (-7.739, 2.2197) (-7.7816, 2.2331) (-7.8242, 2.2464) (-7.8668, 2.2595) (-7.9094, 2.2725) (-7.952, 2.2852) (-7.9947, 2.2978) (-8.0373, 2.3102) (-8.08, 2.3224) (-8.1227, 2.3344) (-8.1653, 2.3463) (-8.208, 2.3579) (-8.2507, 2.3694) (-8.2934, 2.3807) (-8.3361, 2.3918) (-8.3789, 2.4027) (-8.4216, 2.4133) (-8.4643, 2.4238) (-8.5071, 2.4341) (-8.5498, 2.4442) (-8.5926, 2.4541) (-8.6353, 2.4638) (-8.6781, 2.4732) (-8.7209, 2.4825) (-8.7636, 2.4915) (-8.8064, 2.5003) (-8.8492, 2.5089) (-8.892, 2.5173) (-8.928, 2.5241) (-8.9555, 2.5292) (-8.9744, 2.5326) (-8.9847, 2.5345) (-8.9865, 2.5348) knots -1 -1 -1 -1 -1 -1 -0.985714 -0.971429 -0.957143 -0.942857 -0.928571 -0.914286 -0.9 -0.885714 -0.871429 -0.857143 -0.842857 -0.828571 -0.814286 -0.8 -0.785714 -0.771429 -0.757143 -0.742857 -0.728571 -0.714286 -0.7 -0.685714 -0.671429 -0.657143 -0.642857 -0.628571 -0.614286 -0.6 -0.585714 -0.571429 -0.557143 -0.542857 -0.528571 -0.514286 -0.5 -0.485714 -0.471429 -0.457143 -0.442857 -0.428571 -0.414286 -0.4 -0.385714 -0.371429 -0.357143 -0.354152 -0.354152 -0.354152 -0.354152 -0.354152 -0.354152
  spline S135 degree 3 poles (-9.3954, 2.9785) (-9.3891, 2.9137) (-9.3702, 2.8507) (-9.3093, 2.7356) (-9.2679, 2.6845) (-9.1848, 2.6153) (-9.1483, 2.5921) (-9.0702, 2.5556) (-9.0289, 2.5425) (-8.9865, 2.5348) knots 0 0 0 0 0.019532 0.019532 0.039064 0.039064 0.051994 0.051994 0.064924 0.064924 0.064924 0.064924
  arc A68 (-9.3954, 2.9785) -> (-9.4037, 3.0628) centre (-40, 0) ccw
  spline S136 degree 3 poles (-9.0895, 3.5778) (-9.15, 3.5539) (-9.2054, 3.5185) (-9.2993, 3.4283) (-9.3371, 3.3745) (-9.3809, 3.2755) (-9.3931, 3.234) (-9.4067, 3.1489) (-9.408, 3.1057) (-9.4037, 3.0628) knots 0 0 0 0 0.019532 0.019532 0.039064 0.039064 0.051994 0.051994 0.064924 0.064924 0.064924 0.064924